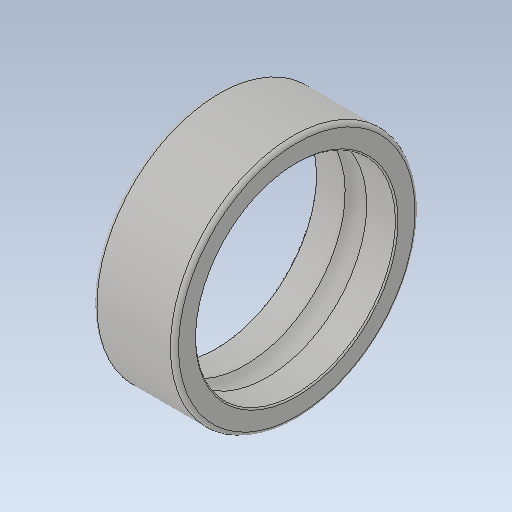
# Autodesk Inventor part: SKF_W 617/3_PART2
Saved by Autodesk Inventor 2021.4 (Build 254397000, 397)
## iProperties
Created: 2022-07-13
Part Number: SKF_W 617/3_PART2
Material: Generic
Catalog Web Link: www.cadenas.de
Description: -Deep groove ball bearings
Vendor: SKF
Document SubType Name: Modeling
Designer: psAdmin
Manufacturer: SKF
Mass: 0.0181787 g
Surface Area: 0.86249 cm^2
Volume: 0.0181787 cm^3
Density: 1 g/cm^3
Appearance: PSOLRGB-175-175-175
Category: PARTsolutions
Company: SKF
PSOL_IDENT_0: {$CADENAS_DATA/23d-libs/skf/bearings_units_and_housings/ball_bearings/deep_groove_ball_bearings/bb1_
PSOL_IDENT_1: 001_101.prj},201 {VTYP=3D},{NB=SKF_W 617/3_PART2},{LINA=SKF_W 617/3_PART2},{NN=BB1_001_101_PART2},{N
PSOL_IDENT_2: OPRJ=TRUE},{DATE=08.07.2022 10:24:27},{GEOMDATE=04.07.2022 10:54:51},{VERSION=},{LINEID=18990},{WBVA
PSOL_IDENT_3: R=},{WBNUMERIC=}  {NB=SKF_W 617/3_PART2},{LINA=SKF_W 617/3_PART2},{KT=DUMMY},{DESIGNATION=W 617/3},{
PSOL_IDENT_4: R12=0.10},{DD=3.000},{D=6.000},{B=2.000},{C=},{CX=},{CXX=},{CA=0.000},{XXVARIANT=},{XXDESIGN=Single
PSOL_IDENT_5: row stainless steel},{XXSEALING=No seals},{DESIGN=dgbbw},{DESIGNIR=dgbbw},{VARIANT=},{DD1=3.70},{DD2=
PSOL_IDENT_6: },{DD2X=},{DD2A=0.00},{D1=4.90},{D1X=0.00},{D2=},{D2A=0.00},{D3=},{D3X=},{D3A=0.000},{D4=},{HH=0.000
PSOL_IDENT_7: },{BB=0.000},{BBX=},{BBA=0.000},{FF=},{R0MAX=0.000},{R0=0.000},{PITCH=4.30},{DW=0.800},{DDAMIN=3.600
PSOL_IDENT_8: },{DDAMAX=0.000},{DDBMIN=0.000},{DDBMAX=0.000},{DBMIN=0.000},{DAMAX=5.200},{BBAMIN=0.000},{CAMAX=0.0
PSOL_IDENT_9: 00},{RAMAX=0.100},{LOAD1=0.117},{LOAD2=0.036},{LOAD3=0.002},{SPEED1=170000},{SPEED2=110000},{KR=0.01
PSOL_IDENT_10: 5},{F0=7.100},{Z=8},{II=1},{MASS=0.000},{BEARING=W 617/3},{RING=},{HELP=0.550},{HELP2=0.550},{DD1ALG=
PSOL_IDENT_11: 1.850},{YALG=1.850},{PITCH1=4.300},{DW1=0.800},{YALG1=2.450},{HALG1=0.550},{SH=1.850},{CU=0.240},{HA
PSOL_IDENT_12: LG=0.35},{B1=0},{SHIELDHELP=1},{D4A=0.000},{FFA=0.000},{RS1=},{HELP3=0}
NB: SKF_W 617/3_PART2
NT: Deep groove ball bearings
NBSYN: SKF_$DESIGNATION._PART2
LINA: SKF_W 617/3_PART2
CATALOG: SKF
DESIGNATION: W 617/3
R12: 0.1
DD: 3
D: 6
B: 2
XXDESIGN: Single row stainless steel
XXSEALING: No seals
LOAD1: 0.117
LOAD2: 0.036
LOAD3: 0.002
SPEED1: 170000
SPEED2: 110000
BEARING: W 617/3
SUPPLIER: SKF
ARTICLENO: SKF_W 617/3_PART2
BOMINFO: SKF_W 617/3_PART2
CREATOR: CADENAS GmbH
Title: SKF_W 617/3_PART2
Author: Cadenas PARTsolutions
Comments: Deep groove ball bearings
Autodesk Inventor part; units mm, degrees
ref_plane "YZ Plane" through (0, 0, 0) normal (1, 0, 0) x (0, 1, 0)
ref_plane "XZ Plane" through (0, 0, 0) normal (0, 1, 0) x (-1, 0, 0)
ref_plane "XY Plane" through (0, 0, 0) normal (0, 0, 1) x (1, 0, 0)
sketch "Sketch_7" plane through (0, 0, 0) normal (0, 0, 1) x (1, 0, 0)
  line L0 (2, 0) -> (-2, 0)
  arc A0 (0, 2.4833) -> (0.0333, 2.45) centre (0.0333, 2.4833) ccw
  line L1 (0.0333, 2.45) -> (0.7354, 2.45)
  arc A1 (1.2646, 2.45) -> (0.7354, 2.45) centre (1, 2.15) ccw
  line L2 (1.2646, 2.45) -> (1.9667, 2.45)
  arc A2 (1.9667, 2.45) -> (2, 2.4833) centre (1.9667, 2.4833) ccw
  line L3 (2, 2.4833) -> (2, 2.9)
  arc A3 (2, 2.9) -> (1.9, 3) centre (1.9, 2.9) ccw
  line L4 (1.9, 3) -> (0.1, 3)
  arc A4 (0.1, 3) -> (0, 2.9) centre (0.1, 2.9) ccw
  line L5 (0, 2.9) -> (0, 2.4833)
  constraints: 12 end point, 10 point on circle, 5 centre point
revolve "Revolution1" add sketch "Sketch_7" angle 360 about axis through (2, 0, 0) along (1, 0, 0)
body "Solid1"
